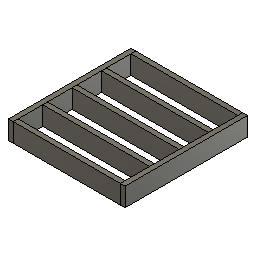
spices_shelfs v7 (Autodesk Fusion 360 design; units mm, degrees)
Autodesk Fusion 360 part; units mm, degrees
sketch "Sketch1" plane through (0, 0, 0) normal (0, 0, 1) x (1, 0, 0) in component "Base"
  line L0 (0, 0) -> (400, 0)
  line L1 (400, 0) -> (400, 70)
  line L2 (400, 70) -> (0, 70)
  line L3 (0, 70) -> (0, 0)
  dimension "d5" = 400
  dimension "d6" = 70
  constraint horizontal L0
  constraint vertical L1
  constraint horizontal L2
  constraint vertical L3
  constraint coincident L0.start L3.end
  measures "d5" distance of L0.start L0.end
  measures "d6" distance of L0.end L1.end
extrude "Extrude1" add sketch "Sketch1" along normal blind 18 makes body 1 in component "Base"
sketch "Sketch1 (2)" plane through (0, 0, 0) normal (-1, 0, 0) x (0, 0, 1) in component "wall"
  line L0 (0, 70) -> (0, 0)
  line L1 (0, 0) -> (18, 0)
  line L2 (18, 0) -> (18, 70)
  line L3 (18, 70) -> (0, 70)
  line L4 (0, 70) -> (458, 70)
  line L5 (458, 70) -> (458, 0)
  line L6 (458, 0) -> (0, 0)
  line L7 (0, 0) -> (0, 70)
  dimension "d10" = 458
  constraint horizontal L4
  constraint vertical L5
  constraint horizontal L6
  constraint vertical L7
  constraint coincident L0.start L3.end
  constraint collinear L1 L6
  measures "d10" distance of L0.end L5.end
extrude "Extrude1'" add sketch "Sketch1 (2)" along normal blind 18 separate body makes body 2 in component "wall"
pattern_linear "00000000-0000-0000-0000-000000000000" [suppressed]
component "Base" placed x (1, 0, 0) y (0, 1, 0) z (0, 0, 1) at (124.288, -10.0095, 62.6397)
component "wall" placed x (1, 0, 0) y (0, 1, 0) z (0, 0, 1) at (124.288, -10.0095, 62.6397)
component "wall" placed x (1, 0, 0) y (0, 1, 0) z (0, 0, 1) at (542.288, -10.0095, 62.6397)
component "Base" placed x (1, 0, 0) y (0, 1, 0) z (0, 0, 1) at (124.288, -10.0095, 502.6397)
component "Base" placed x (1, 0, 0) y (0, 1, 0) z (0, 0, 1) at (124.288, -10.0095, 172.6397)
component "Base" placed x (1, 0, 0) y (0, 1, 0) z (0, 0, 1) at (124.288, -10.0095, 282.6397)
component "Base" placed x (1, 0, 0) y (0, 1, 0) z (0, 0, 1) at (124.288, -10.0095, 392.6397)
equation "shelf_depth = 70.00 mm"
equation "shelf_width = 400.00 mm"
equation "shelfs_number = 4"
equation "shelf_height = 92.00 mm"
equation "d5 = shelf_width"
equation "d6 = shelf_depth"
equation "board_thickness = 18.00 mm"
equation "d8 = board_thickness"
equation "d10 = shelfs_number * ( board_thickness + shelf_height ) + board_thickness"
equation "d11 = board_thickness"
equation "d25 = shelfs_number"
equation "d27 = shelf_height + board_thickness"
